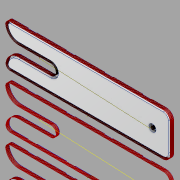
# Autodesk Inventor part: wheel_mount
Saved by Autodesk Inventor 2021.3 (Build 253353000, 353)
## iProperties
Created: 2021-07-08
Part Number: wheel_mount
Material: アルミニウム 6061
Document SubType Name: Modeling
Designer: gisen
Density: 2.7 g/cm^3
Appearance: アルミニウム - フラット
Author: gisen
Autodesk Inventor part; units mm, degrees
ref_plane "YZ Plane" through (0, 0, 0) normal (1, 0, 0) x (0, 1, 0)
ref_plane "XZ Plane" through (0, 0, 0) normal (0, 1, 0) x (-1, 0, 0)
ref_plane "作業平面1" through (0, 0, 0) normal (0, 0, 1) x (1, 0, 0)
sketch "スケッチ2" plane through (0, 0, 0) normal (0, 0, 1) x (1, 0, 0)
  line L0 (110, -57) -> (-40, -57)
  line L1 (-40, -57) -> (-40, -93)
  line L2 (-40, -93) -> (110, -93)
  line L3 (110, -93) -> (110, -57)
  circle A0 centre (0, -75) radius 6 construction
  circle A1 centre (0, -75) radius 75 construction
  point P0 (0, 0)
  dimension "d1" = 150
  dimension "d2" = 18
  dimension "d3" = 18
  dimension "d4" = 40
  dimension "d29" = 110
  constraints: 8 end point, 2 parallel, 1 horizontal, 1 perpendicular, 1 vertical alignment
  measures "d2" distance from line of L0 A0.centre
  measures "d3" distance from line of L2 A0.centre
  measures "d4" distance from line of L1 A0.centre
  measures "d29" distance from line of A0.centre L3
extrude "押し出し1" add sketch "スケッチ2" along normal blind 3
sketch "スケッチ3" plane through (0, 0, 3) normal (0, 0, 1) x (1, 0, 0)
  circle A0 centre (0, -75) radius 6 construction
  circle A1 centre (0, -75) radius 7
  line L0 (0, -68) -> (-38.1, -68) construction
  line L1 (-38.1, -68) -> (-38.1, -82) construction
  line L2 (-38.1, -82) -> (0, -82) construction
  line L3 (0, -82) -> (0, -68) construction
  line L4 (0, -68) -> (-40, -68)
  line L5 (-40, -68) -> (-40, -82)
  line L6 (-40, -82) -> (0, -82)
  line L7 (0, -82) -> (0, -68)
  line L8 (-40, -57) -> (-40, -93) projected
  point P0 (0, 0)
  point P1 (0, -82)
  dimension "d8" = 14
  constraints: 16 end point, 4 horizontal, 4 parallel, 2 perpendicular, 1 coincident, 1 collinear, 1 point on line, 3 other
extrude "押し出し2" cut sketch "スケッチ3" against normal blind 14
fillet "フィレット1" radius 10 2 edges at (-40, -68, 1.5) (-40, -82, 1.5)
ref_plane "作業平面2" through (-40, -75, 0) normal (0, -1, 0) x (1, 0, 0)
sketch "スケッチ4" plane through (0, 0, 3) normal (0, 0, 1) x (1, 0, 0)
  line L0 (-40, -93) -> (110, -93) projected
  line L1 (110, -57) -> (-40, -57) projected
  line L2 (110, -93) -> (110, -57) projected
  point P0 (0, 0)
  point P1 (95, -75)
  dimension "d25" = 15
  dimension "d26" = 36
  dimension "d27" = 18
  measures "d25" distance from line of L2 point (95, -75)
  measures "d26" distance between parallel lines of L0 L1
  measures "d27" distance from line of L1 point (95, -75)
hole "穴1" at (95, -75, 3) direction (0, 0, -1) diameter 6.6 end through all
fillet "フィレット2" radius 5 2 edges at (110, -57, 1.5) (110, -93, 1.5)
fillet "フィレット2" radius 2 2 edges at (-40, -57, 1.5) (-40, -93, 1.5)
ref_plane "作業平面3" through (0, -75, 0) normal (0, 0.7071, 0.7071) x (-1, 0, 0)
equation "\"d3\" = d2"
equation "\"d9\" = d8"
equation "\"d27\" = 0.5 * d26"
